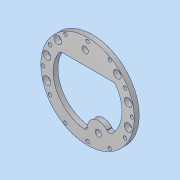
# Autodesk Inventor part: AluminumSealingDiscMidshipsRear
Saved by Autodesk Inventor 2017 (Build 210142000, 142)
## iProperties
Created: 2016-10-25
Part Number: AluminumSealingDiscMidshipsRear
Material: Aluminum 6061
Document SubType Name: Modeling
Designer: techn
Density: 2.7 g/cm^3
Appearance: Aluminum - Flat
Mass: 35.6806 g
Surface Area: 93.6859 cm^2
Volume: 13.215 cm^3
Author: techn
Autodesk Inventor part; units mm, degrees
ref_plane "YZ Plane" through (0, 0, 0) normal (1, 0, 0) x (0, 1, 0)
ref_plane "XZ Plane" through (0, 0, 0) normal (0, 1, 0) x (-1, 0, 0)
ref_plane "XY Plane" through (0, 0, 0) normal (0, 0, 1) x (1, 0, 0)
sketch "Sketch1" plane through (0, 0, 0) normal (0, 0, 1) x (1, 0, 0)
  circle A0 centre (0, 0) radius 45.212
  dimension "d0" = 90.424
  constraints: 1 centre point, 1 coincident
  measures "d0" diameter of A0
extrude "Extrusion1" add sketch "Sketch1" along normal blind 4.7625
sketch "Sketch6" plane through (0, 0, 4.7625) normal (0, 0, 1) x (1, 0, 0)
  circle A0 centre (10.541, -29.7561) radius 3.1242
  point P0 (0, 0)
  dimension "d27" = 6.2484
  dimension "d28" = 29.7561
  dimension "d29" = 10.541
  constraints: 1 centre point
  measures "d27" diameter of A0
  measures "d28" vertical distance of A0.centre point (0, 0)
  measures "d29" horizontal distance of A0.centre point (0, 0)
extrude "Extrusion6" cut sketch "Sketch6" against normal blind 25.4
sketch "Sketch7" plane through (0, 0, 4.7625) normal (0, 0, 1) x (1, 0, 0)
  line L0 (0, 0) -> (21.4313, 37.12)
  line L1 (0, 0) -> (42.8625, 0) construction
  circle A0 centre (21.4313, 37.12) radius 1.7145
  circle A1 centre (-21.4312, 37.12) radius 1.7145
  circle A2 centre (-42.8625, 0) radius 1.7145
  circle A3 centre (-21.4313, -37.12) radius 1.7145
  circle A4 centre (21.4312, -37.12) radius 1.7145
  circle A5 centre (42.8625, 0) radius 1.7145
  dimension "d32" = 42.8625
  dimension "d33" = 60
  dimension "d34" = 3.429
  dimension "d37" = 360
  constraints: 6 centre point, 4 end point, 1 coincident, 1 equal length, 1 horizontal, 13 other
  measures "d32" distance of L0.start L0.end
  measures "d33" angle of L1 L0
  measures "d34" diameter of A0
extrude "Extrusion7" cut sketch "Sketch7" against normal blind 25.4
sketch "Sketch8" plane through (0, 0, 4.7625) normal (0, 0, 1) x (1, 0, 0)
  line L0 (0, 0) -> (0, 41.91)
  circle A0 centre (0, 41.91) radius 1.8415
  circle A1 centre (-36.2951, 20.955) radius 1.8415
  circle A2 centre (-36.2951, -20.955) radius 1.8415
  circle A3 centre (0, -41.91) radius 1.8415
  circle A4 centre (36.2951, -20.955) radius 1.8415
  circle A5 centre (36.2951, 20.955) radius 1.8415
  dimension "d41" = 41.91
  dimension "d42" = 3.683
  dimension "d45" = 360
  constraints: 6 centre point, 2 end point, 1 coincident, 1 vertical, 13 other
  measures "d41" distance of L0.start L0.end
  measures "d42" diameter of A0
extrude "Extrusion8" cut sketch "Sketch8" against normal blind 25.4
sketch "Sketch10" plane through (0, 0, 4.7625) normal (0, 0, 1) x (1, 0, 0)
  line L0 (0, 0) -> (39.3779, 10.5513)
  line L1 (0, 0) -> (40.767, 0) construction
  circle A0 centre (39.3779, 10.5513) radius 3.81
  line L2 (0, 0) -> (0, 16.2318)
  circle A1 centre (39.3779, -10.5513) radius 3.81
  circle A2 centre (-39.3779, 10.5513) radius 3.81
  circle A3 centre (-39.3779, -10.5513) radius 3.81
  line L3 (0, 0) -> (28.8266, 28.8266)
  line L4 (0, 0) -> (40.767, 0) construction
  circle A4 centre (28.8266, 28.8266) radius 3.81
  circle A5 centre (-28.8266, 28.8266) radius 3.81
  dimension "d49" = 40.767
  dimension "d50" = 15
  dimension "d51" = 7.62
  dimension "d68" = 40.767
  dimension "d69" = 45
  dimension "d70" = 7.62
  constraints: 10 end point, 6 centre point, 4 symmetric about line, 2 coincident, 2 equal length, 2 horizontal, 1 vertical, 4 other
  measures "d49" distance of L0.start L0.end
  measures "d50" angle of L1 L0
  measures "d51" diameter of A0
  measures "d68" distance of L0.start L3.end
  measures "d69" angle of L4 L3
  measures "d70" diameter of A4
extrude "Extrusion9" cut sketch "Sketch10" against normal blind 25.4 contours A0 | A1 | A2 | A3
sketch "Sketch11" plane through (0, 0, 4.7625) normal (0, 0, 1) x (1, 0, 0)
  circle A0 centre (-39.3779, 10.5513) radius 3.81 projected
  circle A1 centre (39.3779, 10.5513) radius 3.81 projected
  circle A2 centre (39.3779, -10.5513) radius 3.81 projected
  circle A3 centre (-39.3779, -10.5513) radius 3.81 projected
  circle A4 centre (36.2951, -20.955) radius 1.8415 projected
  circle A5 centre (-36.2951, -20.955) radius 1.8415 projected
  circle A6 centre (0, 41.91) radius 1.8415 projected
  circle A7 centre (-36.2951, 20.955) radius 1.8415 projected
  circle A8 centre (0, -41.91) radius 1.8415 projected
  circle A9 centre (36.2951, 20.955) radius 1.8415 projected
  circle A10 centre (21.4312, -37.12) radius 1.7145 projected
  circle A11 centre (-42.8625, 0) radius 1.7145 projected
  circle A12 centre (21.4313, 37.12) radius 1.7145 projected
  circle A13 centre (-21.4312, 37.12) radius 1.7145 projected
  circle A14 centre (-21.4313, -37.12) radius 1.7145 projected
  circle A15 centre (42.8625, 0) radius 1.7145 projected
  circle A16 centre (10.541, -29.7561) radius 3.1242 projected
  circle A17 centre (0, 0) radius 45.212 projected
  circle A18 centre (0, 0) radius 20.6375
  dimension "d54" = 41.275
  constraints: 1 centre point, 1 coincident
  measures "d54" diameter of A18
extrude "Extrusion10" cut sketch "Sketch11" against normal blind 25.4 contours A18
sketch "Sketch12" plane through (0, 0, 4.7625) normal (0, 0, 1) x (1, 0, 0)
  circle A0 centre (0, 0) radius 20.6375 projected
  circle A1 centre (-39.3779, 10.5513) radius 3.81 projected
  circle A2 centre (39.3779, 10.5513) radius 3.81 projected
  circle A3 centre (39.3779, -10.5513) radius 3.81 projected
  circle A4 centre (-39.3779, -10.5513) radius 3.81 projected
  circle A5 centre (36.2951, -20.955) radius 1.8415 projected
  circle A6 centre (-36.2951, -20.955) radius 1.8415 projected
  circle A7 centre (0, 41.91) radius 1.8415 projected
  circle A8 centre (-36.2951, 20.955) radius 1.8415 projected
  circle A9 centre (0, -41.91) radius 1.8415 projected
  circle A10 centre (36.2951, 20.955) radius 1.8415 projected
  circle A11 centre (21.4312, -37.12) radius 1.7145 projected
  circle A12 centre (-42.8625, 0) radius 1.7145 projected
  circle A13 centre (21.4313, 37.12) radius 1.7145 projected
  circle A14 centre (-21.4312, 37.12) radius 1.7145 projected
  circle A15 centre (-21.4313, -37.12) radius 1.7145 projected
  circle A16 centre (42.8625, 0) radius 1.7145 projected
  circle A17 centre (10.541, -29.7561) radius 3.1242 projected
  circle A18 centre (0, 0) radius 45.212 projected
  circle A19 centre (0, 0) radius 33.3375
  line L0 (0, 0) -> (0, -33.3375)
  line L1 (0, 0) -> (10.541, -29.7561)
  line L2 (0, 0) -> (20.9859, -25.9033)
  line L3 (0, -20.6375) -> (0, -33.3375)
  line L4 (12.9913, -16.0354) -> (20.9859, -25.9033)
  arc A20 (0, -20.6375) -> (12.9913, -16.0354) centre (0, 0) ccw
  arc A21 (0, -33.3375) -> (20.9859, -25.9033) centre (0, 0) ccw
  dimension "d57" = 66.675
  constraints: 10 end point, 8 point on circle, 3 centre point, 3 point on line, 2 collinear, 2 concentric, 1 coincident, 1 symmetric about line, 1 vertical
  measures "d57" diameter of A19
extrude "Extrusion11" cut sketch "Sketch12" against normal blind 25.4 contours A0 L0 A19 L2
sketch "Sketch13" plane through (0, 0, 4.7625) normal (0, 0, 1) x (1, 0, 0)
  line L0 (20.9859, -25.9033) -> (12.9913, -16.0354) projected
  arc A0 (0, -20.6375) -> (12.9913, -16.0354) centre (0, 0) ccw projected
  line L1 (0, -20.6375) -> (0, -33.3375) projected
  arc A1 (20.9859, -25.9033) -> (0, -33.3375) centre (0, 0) ccw projected
  circle A2 centre (-39.3779, 10.5513) radius 3.81 projected
  circle A3 centre (39.3779, 10.5513) radius 3.81 projected
  circle A4 centre (39.3779, -10.5513) radius 3.81 projected
  circle A5 centre (-39.3779, -10.5513) radius 3.81 projected
  circle A6 centre (36.2951, -20.955) radius 1.8415 projected
  circle A7 centre (-36.2951, -20.955) radius 1.8415 projected
  circle A8 centre (0, 41.91) radius 1.8415 projected
  circle A9 centre (-36.2951, 20.955) radius 1.8415 projected
  circle A10 centre (0, -41.91) radius 1.8415 projected
  circle A11 centre (36.2951, 20.955) radius 1.8415 projected
  circle A12 centre (21.4312, -37.12) radius 1.7145 projected
  circle A13 centre (-42.8625, 0) radius 1.7145 projected
  circle A14 centre (21.4313, 37.12) radius 1.7145 projected
  circle A15 centre (-21.4312, 37.12) radius 1.7145 projected
  circle A16 centre (-21.4313, -37.12) radius 1.7145 projected
  circle A17 centre (42.8625, 0) radius 1.7145 projected
  circle A18 centre (10.541, -29.7561) radius 3.1242 projected
  circle A19 centre (0, 0) radius 45.212 projected
  circle A20 centre (10.541, -29.7561) radius 10.541
  arc A21 (18.7314, -23.1206) -> (0, -29.7561) centre (10.541, -29.7561) ccw
  constraints: 4 point on circle, 2 centre point, 2 concentric, 2 point on line, 1 coincident, 1 tangent
extrude "Extrusion12" cut sketch "Sketch13" against normal blind 25.4 contours L0 A0 L1 A1 | A20 L1 A0 L0
fillet "Fillet2" radius 3.175 2 edges at (20.9859, -25.9033, 2.3813) (0, -33.3375, 2.3813)
sketch "Sketch14" plane through (0, 0, 4.7625) normal (0, 0, 1) x (1, 0, 0)
  circle A0 centre (0, 0) radius 45.212 projected
  circle A1 centre (10.541, -29.7561) radius 3.1242 projected
  circle A2 centre (42.8625, 0) radius 1.7145 projected
  circle A3 centre (-21.4313, -37.12) radius 1.7145 projected
  circle A4 centre (-21.4312, 37.12) radius 1.7145 projected
  circle A5 centre (21.4313, 37.12) radius 1.7145 projected
  circle A6 centre (-42.8625, 0) radius 1.7145 projected
  circle A7 centre (21.4312, -37.12) radius 1.7145 projected
  circle A8 centre (36.2951, 20.955) radius 1.8415 projected
  circle A9 centre (0, -41.91) radius 1.8415 projected
  circle A10 centre (-36.2951, 20.955) radius 1.8415 projected
  circle A11 centre (0, 41.91) radius 1.8415 projected
  circle A12 centre (-36.2951, -20.955) radius 1.8415 projected
  circle A13 centre (36.2951, -20.955) radius 1.8415 projected
  circle A14 centre (-39.3779, -10.5513) radius 3.81 projected
  circle A15 centre (39.3779, -10.5513) radius 3.81 projected
  circle A16 centre (39.3779, 10.5513) radius 3.81 projected
  circle A17 centre (-39.3779, 10.5513) radius 3.81 projected
  arc A18 (18.7314, -23.1206) -> (0, -29.7561) centre (10.541, -29.7561) ccw projected
  line L0 (0, -29.7561) -> (0, -29.9949) projected
  arc A19 (-3.5092, -33.1523) -> (0, -29.9949) centre (-3.175, -29.9949) ccw projected
  arc A20 (23.5959, -23.5504) -> (-3.5092, -33.1523) centre (0, 0) ccw projected
  arc A21 (18.8817, -23.3061) -> (23.5959, -23.5504) centre (21.3487, -21.3075) ccw projected
  line L1 (18.8817, -23.3061) -> (18.7314, -23.1206) projected
  line L2 (26.4289, 20.32) -> (-26.4289, 20.32)
  dimension "d64" = 20.32
  constraints: 2 end point, 2 point on circle, 1 horizontal
  measures "d64" distance from line of L2 point (0, 0)
extrude "Extrusion13" add sketch "Sketch14" against normal up to surface (4.7625 mm away) contours L2 A20
fillet "Fillet3" radius 3.175 2 edges at (-26.4289, 20.32, 2.3813) (26.4289, 20.32, 2.3813)
extrude "Extrusion14" cut sketch "Sketch10" against normal blind 25.4 contours A4 | A5
sketch "Sketch16" plane through (0, 0, 4.7625) normal (0, 0, 1) x (1, 0, 0)
  circle A0 centre (-2.286, 33.655) radius 3.1242
  point P0 (0, 0)
  dimension "d73" = 6.2484
  dimension "d74" = 2.286
  dimension "d75" = 33.655
  constraints: 1 centre point
  measures "d73" diameter of A0
  measures "d74" horizontal distance of A0.centre point (0, 0)
  measures "d75" vertical distance of point (0, 0) A0.centre
extrude "Extrusion15" cut sketch "Sketch16" against normal through all
body "Solid1"
